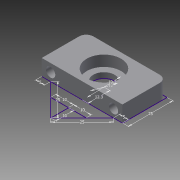
# Autodesk Inventor part: bearing_holder_corner_tb
Saved by Autodesk Inventor 2015 (Build 190159000, 159)
## iProperties
Created: 2018-01-11
Part Number: bearing_holder_corner_tb
Material: Generic
Document SubType Name: Modeling
Designer: Anshul
Density: 1 g/cm^3
Appearance: Default
Author: Anshul
Autodesk Inventor part; units mm, degrees
ref_plane "YZ Plane" through (0, 0, 0) normal (1, 0, 0) x (0, 1, 0)
ref_plane "XZ Plane" through (0, 0, 0) normal (0, 1, 0) x (-1, 0, 0)
ref_plane "XY Plane" through (0, 0, 0) normal (0, 0, 1) x (1, 0, 0)
sketch "Sketch1" plane through (0, 0, 0) normal (0, 1, 0) x (-1, 0, 0)
  line L0 (0, 0) -> (0, -10)
  line L1 (0, -10) -> (10, -10)
  line L2 (10, -10) -> (0, 0)
  line L3 (0, -10) -> (-10, -10)
  line L4 (-10, -10) -> (0, 0)
  line L5 (0, 0) -> (17.6777, -17.6777)
  line L6 (0, 0) -> (-17.6777, -17.6777)
  line L7 (-17.6777, -17.6777) -> (17.6777, -17.6777)
  line L8 (0, -17.6777) -> (0, -29.9777)
  circle A0 centre (0, -29.9777) radius 9.65
  circle A1 centre (0, -29.9777) radius 6
  line L9 (17.6777, -17.6777) -> (22.6777, -17.6777)
  line L10 (-17.6777, -17.6777) -> (-22.6777, -17.6777)
  line L11 (-22.6777, -17.6777) -> (-22.6777, -42.6777)
  line L12 (-22.6777, -42.6777) -> (22.6777, -42.6777)
  line L13 (22.6777, -42.6777) -> (22.6777, -17.6777)
  dimension "d0" = 10
  dimension "d1" = 10
  dimension "d2" = 10
  dimension "d3" = 25
  dimension "d4" = 25
  dimension "d5" = 12.3
  dimension "d6" = 19.3
  dimension "d7" = 12
  dimension "d8" = 5
  dimension "d9" = 5
  dimension "d10" = 25
  constraints: 28 end point, 3 perpendicular, 3 point on line, 3 vertical, 2 centre point, 2 coincident, 2 horizontal, 1 midpoint
  measures "d0" distance of L0.start L0.end
  measures "d1" distance of L0.end L1.end
  measures "d2" distance of L0.end L3.end
  measures "d3" distance of L0.start L5.end
  measures "d4" distance of L0.start L6.end
  measures "d5" distance of L8.start L8.end
  measures "d6" diameter of A0
  measures "d7" diameter of A1
  measures "d8" distance of L5.end L9.end
  measures "d9" distance of L6.end L10.end
  measures "d10" distance of L10.end L11.end
extrude "Extrusion1" add sketch "Sketch1" along normal blind 3 contours A0
extrude "Extrusion2" add sketch "Sketch1" along normal blind 9 contours L9 L13 L12 L11 L10 L7
sketch "Sketch2" plane through (-22.6777, 0, -17.6777) normal (0, 0, 1) x (1, 0, 0)
  line L0 (0, 0) -> (0, 9)
  line L1 (0, 4.5) -> (5, 4.5)
  line L2 (45.3553, 9) -> (45.3553, 0)
  line L3 (45.3553, 4.5) -> (40.3553, 4.5)
  circle A0 centre (5, 4.5) radius 2.6
  circle A1 centre (40.3553, 4.5) radius 2.6
  point P0 (22.6777, 0)
  dimension "d15" = 5
  dimension "d16" = 5
  dimension "d17" = 5.2
  dimension "d18" = 5.2
  constraints: 8 end point, 2 centre point, 2 coincident, 2 midpoint, 2 vertical, 1 horizontal, 1 point on line
  measures "d15" distance of L1.start L1.end
  measures "d16" distance of L3.start L3.end
  measures "d17" diameter of A0
  measures "d18" diameter of A1
extrude "Extrusion3" cut sketch "Sketch2" against normal blind 26
fillet "Fillet1" radius 4 2 edges at (22.6777, 4.5, -42.6777) (-22.6777, 4.5, -42.6777)
body "Solid1"
